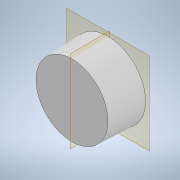
# Autodesk Inventor part: 20_Cube_Insert_VCAmount2_inside_2
Saved by Autodesk Inventor 2022.3 (Build 263350000, 350)
## iProperties
Created: 2022-05-25
Part Number: 20_Cube_Insert_VCAmount2_inside_2
Material: Generic
Document SubType Name: Modeling
Designer: bingoeleda
Density: 1 g/cm^3
Appearance: Default
Author: bingoeleda
Autodesk Inventor part; units mm, degrees
ref_plane "XZ Plane" through (0, 0, 0) normal (0, 1, 0) x (-1, 0, 0)
sketch "Sketch6" plane through (0, 0, 0) normal (0, 0, 1) x (1, 0, 0)
  circle A0 centre (0, 0) radius 6.25
  dimension "d34" = 12.5
  constraints: 1 centre point, 1 coincident
  measures "d34" diameter of A0
extrude "Extrusion4" add sketch "Sketch6" along normal blind 6 draft -2.5
body "Solid2"
